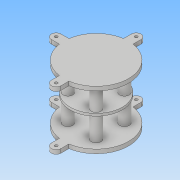
# Autodesk Inventor part: Height_upgrade
Saved by Autodesk Inventor 2019.4 (Build 234330000, 330)
## iProperties
Created: 2019-08-01
Part Number: Height_upgrade
Material: Generic
Document SubType Name: Modeling
Designer: leode
Density: 1 g/cm^3
Appearance: Default
Author: leode
Autodesk Inventor part; units mm, degrees
note: some values were not read from the file. Chosen so that the rebuilt part matches the saved one: sketch regions of "Extrusion1".
ref_plane "YZ Plane" through (0, 0, 0) normal (1, 0, 0) x (0, 1, 0)
ref_plane "XZ Plane" through (0, 0, 0) normal (0, 1, 0) x (-1, 0, 0)
ref_plane "XY Plane" through (0, 0, 0) normal (0, 0, 1) x (1, 0, 0)
sketch "Sketch1" plane through (0, 0, 0) normal (0, 1, 0) x (-1, 0, 0)
  circle A0 centre (0, 0) radius 40.5
  circle A1 centre (0, 0) radius 39
  line L0 (0, 50) -> (0, -50) construction
  arc A2 (6, 50) -> (-6, 50) centre (0, 50) ccw
  arc A3 (-6, -50) -> (6, -50) centre (0, -50) ccw
  line L1 (0, 0) -> (50, 0) construction
  arc A4 (50, -6) -> (50, 6) centre (50, 0) ccw
  line L2 (0, 0) -> (50, 0) construction
  line L3 (50, 6) -> (40.0531, 6)
  line L4 (40.0531, -6) -> (50, -6)
  line L5 (6, 40.0531) -> (6, 50)
  line L6 (-6, 50) -> (-6, 40.0531)
  line L7 (-6, -40.0531) -> (-6, -50)
  line L8 (6, -50) -> (6, -40.0531)
  circle A5 centre (50, 0) radius 1.75
  circle A6 centre (0, -50) radius 1.75
  circle A7 centre (0, 50) radius 1.75
  point P0 (25, 0)
  dimension "d0" = 81
  dimension "d1" = 78
  dimension "d2" = 100
  dimension "d3" = 12
  dimension "d4" = 50
  dimension "d5" = 50
  dimension "d6" = 0
  dimension "d7" = 12
  dimension "d8" = 3.5
  dimension "d9" = 3.5
  dimension "d10" = 3.5
  constraints: 22 end point, 12 point on circle, 10 tangent, 8 centre point, 5 coincident, 5 parallel, 2 horizontal, 2 midpoint, 1 collinear, 1 vertical
  measures "d0" diameter of A0
  measures "d1" diameter of A1
  measures "d2" distance of L0.start L0.end
  measures "d3" diameter of A3
  measures "d4" distance of point (0, 0) L0.start
  measures "d5" distance of L1.start L1.end
  measures "d6" distance between parallel lines of L1 L2
  measures "d7" diameter of A4
  measures "d8" diameter of A5
  measures "d9" diameter of A6
  measures "d10" diameter of A7
extrude "Extrusion1" add sketch "Sketch1" along normal blind 5 contours A0 | A0 L3 A4 L4 | A0 L6 A2 L5 | L8 A3 L7 A0 | A1
sketch "Sketch2" plane through (0, 0, 0) normal (0, -1, 0) x (1, 0, 0)
  line L0 (0, 0) -> (-17.6777, -17.6777)
  line L1 (0, 0) -> (25, 0) construction
  circle A0 centre (-17.6777, -17.6777) radius 6
  circle A1 centre (17.6777, -17.6777) radius 6
  circle A2 centre (17.6777, 17.6777) radius 6
  circle A3 centre (-17.6777, 17.6777) radius 6
  circle A4 centre (17.6777, -17.6777) radius 2
  circle A5 centre (-17.6777, -17.6777) radius 2
  circle A6 centre (17.6777, 17.6777) radius 2
  circle A7 centre (-17.6777, 17.6777) radius 2
  dimension "d13" = 25
  dimension "d14" = 135
  dimension "d15" = 12
  dimension "d18" = 360
  dimension "d22" = 4
  dimension "d23" = 4
  dimension "d24" = 4
  dimension "d25" = 4
  constraints: 8 centre point, 5 coincident, 4 end point, 1 equal length, 1 horizontal, 9 other
  measures "d13" distance of L0.start L0.end
  measures "d14" angle of L0 L1
  measures "d15" diameter of A0
  measures "d22" diameter of A4
  measures "d23" diameter of A5
  measures "d24" diameter of A6
  measures "d25" diameter of A7
extrude "Extrusion2" add sketch "Sketch2" along normal blind 30
sketch "Sketch3" plane through (-17.6777, -30, 17.6777) normal (0, -1, 0) x (1, 0, 0)
  circle A0 centre (17.6777, -17.6777) radius 32.5
  dimension "d26" = 65
  constraints: 1 centre point, 1 coincident
  measures "d26" diameter of A0
extrude "Extrusion3" add sketch "Sketch3" along normal blind 3
sketch "Sketch4" plane through (0, -33, 0) normal (0, -1, 0) x (1, 0, 0)
  circle A0 centre (17.6777, 17.6777) radius 6 projected
  circle A1 centre (17.6777, 17.6777) radius 2 projected
  circle A2 centre (17.6777, -17.6777) radius 2 projected
  circle A3 centre (17.6777, -17.6777) radius 6 projected
  circle A4 centre (-17.6777, 17.6777) radius 2 projected
  circle A5 centre (-17.6777, 17.6777) radius 6 projected
  circle A6 centre (-17.6777, -17.6777) radius 2 projected
  circle A7 centre (-17.6777, -17.6777) radius 6 projected
  point P0 (0, 0)
extrude "Extrusion4" add sketch "Sketch4" along normal blind 30
sketch "Sketch5" plane through (17.6777, -63, -17.6777) normal (0, -1, 0) x (1, 0, 0)
  circle A0 centre (0, 35.3553) radius 6 projected
  circle A1 centre (-35.3553, 0) radius 6 projected
  circle A2 centre (0, 0) radius 6 projected
  circle A3 centre (-35.3553, 35.3553) radius 6 projected
  circle A4 centre (-67.6777, 17.6777) radius 1.75 projected
  circle A5 centre (-17.6777, -32.3223) radius 1.75 projected
  circle A6 centre (-17.6777, 67.6777) radius 1.75 projected
  arc A7 (-23.6777, -32.3223) -> (-11.6777, -32.3223) centre (-17.6777, -32.3223) ccw projected
  line L0 (-11.6777, -22.3754) -> (-11.6777, -32.3223) projected
  arc A8 (-11.6777, -22.3754) -> (-11.6777, 57.7308) centre (-17.6777, 17.6777) ccw projected
  line L1 (-11.6777, 67.6777) -> (-11.6777, 57.7308) projected
  arc A9 (-11.6777, 67.6777) -> (-23.6777, 67.6777) centre (-17.6777, 67.6777) ccw projected
  line L2 (-23.6777, 57.7308) -> (-23.6777, 67.6777) projected
  arc A10 (-23.6777, 57.7308) -> (-57.7308, 23.6777) centre (-17.6777, 17.6777) ccw projected
  line L3 (-67.6777, 23.6777) -> (-57.7308, 23.6777) projected
  arc A11 (-67.6777, 23.6777) -> (-67.6777, 11.6777) centre (-67.6777, 17.6777) ccw projected
  line L4 (-57.7308, 11.6777) -> (-67.6777, 11.6777) projected
  arc A12 (-57.7308, 11.6777) -> (-23.6777, -22.3754) centre (-17.6777, 17.6777) ccw projected
  line L5 (-23.6777, -32.3223) -> (-23.6777, -22.3754) projected
extrude "Extrusion5" add sketch "Sketch5" along normal blind 5 contours A0 | A1 | A2 | A3 | L5 A12 L4 A11 L3 A10 L2 A9 L1 A8 L0 A7
body "Solid1"
